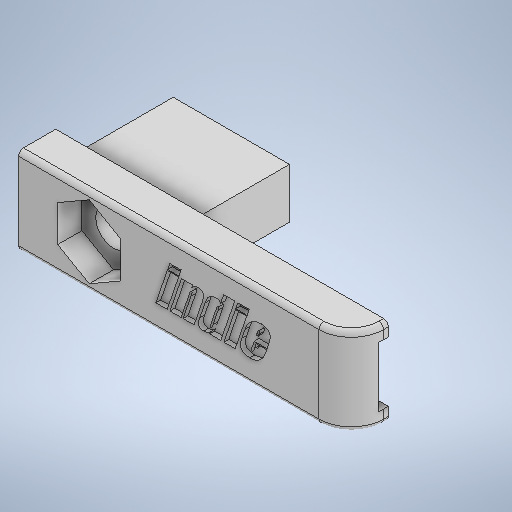
# Autodesk Inventor part: stereotax_holder_side
Saved by Autodesk Inventor 2025 (Build 290162000, 162)
## iProperties
Created: 2023-10-03
Part Number: stereotax_holder_side
Material: Generic
Document SubType Name: Modeling
Designer: mmelin
Density: 1 g/cm^3
Appearance: Default
Author: mmelin
Autodesk Inventor part; units mm, degrees
ref_plane "YZ Plane" through (0, 0, 0) normal (1, 0, 0) x (0, 1, 0)
ref_plane "XZ Plane" through (0, 0, 0) normal (0, 1, 0) x (-1, 0, 0)
ref_plane "XY Plane" through (0, 0, 0) normal (0, 0, 1) x (1, 0, 0)
sketch "Sketch1" plane through (0, 0, 0) normal (0, 0, 1) x (1, 0, 0)
  line L0 (-6.6, -4.4) -> (-23.2373, -4.4) projected
  line L1 (-23.2373, 1) -> (-6.6, 1) projected
  line L2 (-4.6226, -4.4) -> (-25.2226, -4.4)
  line L3 (-25.2226, -4.4) -> (-25.2226, 1)
  line L4 (-25.2226, 1) -> (-4.6226, 1)
  line L5 (-4.6226, 1) -> (-4.6226, -4.4)
  line L6 (-11.6, -0.9) -> (-11.6, -3.4) projected
  line L7 (-4.6226, 0.16) -> (-4.6226, -3.56) projected
  line L8 (-4.6226, 0.16) -> (-15, 0.16) projected
  line L9 (-15, 0.16) -> (-15, -3.56) projected
  line L10 (-15, -3.56) -> (-4.6226, -3.56) projected
  point P0 (0, 0)
  dimension "d1" = 20.6
  dimension "d36" = 0
  constraints: 8 end point, 2 collinear, 2 parallel, 1 horizontal, 1 perpendicular
  measures "d1" distance between parallel lines of L3 L5
  measures "d36" distance between parallel lines of L7 L5
extrude "Extrusion1" add sketch "Sketch1" along normal blind 1.7
sketch "Sketch2" plane through (0, 0, 0) normal (0, 0, -1) x (-1, 0, 0)
  line L0 (4.6226, 0.16) -> (4.6226, -3.56) projected
  line L1 (4.6226, 0.16) -> (15, 0.16) projected
  line L2 (15, 0.16) -> (15, -3.56) projected
  line L3 (15, -3.56) -> (4.6226, -3.56) projected
  line L4 (25.2226, -4.4) -> (4.6226, -4.4) projected
  line L5 (25.2226, 1) -> (25.2226, -4.4) projected
  line L6 (8.5501, -0.0891) -> (8.5501, -3.1391) projected
  line L7 (25.2226, -4.4) -> (4.6226, -4.4) projected
  line L8 (4.6226, -4.4) -> (4.6226, 1) projected
  line L9 (4.6226, 1) -> (25.2226, 1) projected
  line L10 (25.2226, 1) -> (25.2226, -4.4) projected
  line L11 (11.8, -2.35) -> (15, -2.35) projected
  line L12 (11.8, -1.05) -> (11.8, -2.35) projected
  line L13 (15, -1.05) -> (11.8, -1.05) projected
  point P0 (0, 0)
extrude "Extrusion2" add sketch "Sketch2" along normal blind 0.6 contours L8 L9 L5 L4 L3 L2 L1 | L2 L11 L12 L13
fillet "Fillet1" radius 2 1 edges at (-4.6226, -1.7, 1.7)
sketch "Sketch4" plane through (0, 0, -0.6) normal (0, 0, -1) x (-1, 0, 0)
  line L0 (24.45, -3.25) -> (17.25, -3.25)
  line L1 (17.25, -3.25) -> (17.25, -0.15)
  line L2 (17.25, -0.15) -> (24.45, -0.15)
  line L3 (24.45, -0.15) -> (24.45, -3.25)
  line L4 (24.6, -3.4) -> (24.6, 0) projected
  line L5 (17.1, -3.4) -> (24.6, -3.4) projected
  line L6 (17.1, 0) -> (17.1, -3.4) projected
  line L7 (24.6, 0) -> (17.1, 0) projected
  circle A0 centre (20.85, -1.7) radius 1.1 projected
  circle A1 centre (20.85, -1.7) radius 1.1
  point P0 (0, 0)
  dimension "d14" = 0.15
  dimension "d15" = 0.15
  dimension "d16" = 0.15
  dimension "d17" = 0.15
  constraints: 8 end point, 2 parallel, 1 centre point, 1 coincident, 1 concentric, 1 horizontal, 1 perpendicular
  measures "d14" distance between parallel lines of L7 L2
  measures "d15" distance between parallel lines of L6 L1
  measures "d16" distance between parallel lines of L4 L3
  measures "d17" distance between parallel lines of L5 L0
extrude "Extrusion5" add sketch "Sketch4" along normal blind 6.5 contours L0 L1 L2 L3
sketch "Sketch6" plane through (0, 0, 1.7) normal (0, 0, 1) x (1, 0, 0)
  circle A0 centre (-20.85, -1.7) radius 1.1 projected
  circle A1 centre (-20.85, -1.7) radius 1.1
  point P0 (0, 0)
  constraints: 1 centre point, 1 coincident
extrude "Extrusion7" cut sketch "Sketch6" against normal up to surface (8.8 mm away)
sketch "Sketch7" plane through (0, 0, 1.7) normal (0, 0, 1) x (1, 0, 0)
  circle A0 centre (-20.85, -1.7) radius 1.1 projected
  line L0 (-18.9, -2.8258) -> (-20.85, -3.9517)
  line L1 (-20.85, -3.9517) -> (-22.8, -2.8258)
  line L2 (-22.8, -2.8258) -> (-22.8, -0.5742)
  line L3 (-22.8, -0.5742) -> (-20.85, 0.5517)
  line L4 (-20.85, 0.5517) -> (-18.9, -0.5742)
  line L5 (-18.9, -0.5742) -> (-18.9, -2.8258)
  point P0 (0, 0)
  dimension "d27" = 3.9
  constraints: 12 end point, 1 coincident, 1 vertical, 13 other
  measures "d27" distance between parallel lines of L5 L2
extrude "Extrusion8" cut sketch "Sketch7" against normal blind 1.5
fillet "Fillet2" radius 0.3 6 edges at (-15.9226, 1, 1.7) (-5.2084, 1, 1.1142) (-4.6226, 1, -0.45) (-15.9226, -4.4, 1.7) (-5.2084, -4.4, 1.1142) (-4.6226, -4.4, -0.45)
sketch "Sketch9" plane through (0, 0, 1.7) normal (0, 0, 1) x (1, 0, 0)
  line L0 (-16.8365, -0.3734) -> (-8.2904, -0.3734) construction
  line L1 (-8.2904, -0.3734) -> (-8.2904, -3.0273) construction
  line L2 (-8.2904, -3.0273) -> (-16.8365, -3.0273) construction
  line L3 (-16.8365, -3.0273) -> (-16.8365, -0.3734) construction
  line L4 (-15.3132, -0.819) -> (-16.0253, -2.9134)
  line L5 (-16.0253, -2.9134) -> (-16.726, -2.9134)
  line L6 (-16.726, -2.9134) -> (-16.0139, -0.819)
  line L7 (-16.0139, -0.819) -> (-15.3132, -0.819)
  line L8 (-15.1609, -0.3734) -> (-15.2923, -0.76)
  line L9 (-15.2923, -0.76) -> (-15.993, -0.76)
  line L10 (-15.993, -0.76) -> (-15.8616, -0.3734)
  line L11 (-15.8616, -0.3734) -> (-15.1609, -0.3734)
  line L12 (-14.4412, -0.819) -> (-14.5154, -1.0037)
  spline S0 degree 2 poles (-14.5154, -1.0037) (-14.4716, -0.9028) (-14.2203, -0.7828) (-14.0851, -0.7828) knots 0 0 0 1 2 2 2
  spline S1 degree 2 poles (-14.0851, -0.7828) (-13.9137, -0.7828) (-13.75, -0.9465) (-13.7709, -1.1884) (-13.8623, -1.4568) knots 0 0 0 1 2 3 3 3
  line L13 (-13.8623, -1.4568) -> (-14.3574, -2.9134)
  line L14 (-14.3574, -2.9134) -> (-15.0409, -2.9134)
  line L15 (-15.0409, -2.9134) -> (-14.5516, -1.474)
  spline S2 degree 2 poles (-14.5516, -1.474) (-14.4831, -1.2702) (-14.4792, -1.2055) (-14.5173, -1.2055) knots 0 0 0 1 2 2 2
  spline S3 degree 2 poles (-14.5173, -1.2055) (-14.5592, -1.2055) (-14.6106, -1.2836) (-14.6868, -1.5082) knots 0 0 0 1 2 2 2
  line L16 (-14.6868, -1.5082) -> (-15.1647, -2.9134)
  line L17 (-15.1647, -2.9134) -> (-15.8483, -2.9134)
  line L18 (-15.8483, -2.9134) -> (-15.1361, -0.819)
  line L19 (-15.1361, -0.819) -> (-14.4412, -0.819)
  line L20 (-11.8402, -0.3734) -> (-12.7047, -2.9134)
  line L21 (-12.7047, -2.9134) -> (-13.3882, -2.9134)
  line L22 (-13.3882, -2.9134) -> (-13.3387, -2.7649)
  spline S4 degree 2 poles (-13.3387, -2.7649) (-13.4035, -2.8525) (-13.6453, -2.9496) (-13.7595, -2.9496) knots 0 0 0 1 2 2 2
  spline S5 degree 2 poles (-13.7595, -2.9496) (-13.9137, -2.9496) (-14.087, -2.7859) (-14.0775, -2.5726) (-13.9994, -2.3422) knots 0 0 0 1 2 3 3 3
  line L23 (-13.9994, -2.3422) -> (-13.6757, -1.3921)
  spline S6 degree 2 poles (-13.6757, -1.3921) (-13.5958, -1.1522) (-13.4606, -0.9446) (-13.1731, -0.7828) (-13.015, -0.7828) knots 0 0 0 1 2 3 3 3
  spline S7 degree 2 poles (-13.015, -0.7828) (-12.8951, -0.7828) (-12.7199, -0.8723) (-12.7199, -0.9465) knots 0 0 0 1 2 2 2
  line L24 (-12.7199, -0.9465) -> (-12.5238, -0.3734)
  line L25 (-12.5238, -0.3734) -> (-11.8402, -0.3734)
  spline S8 degree 2 poles (-12.8608, -1.3616) (-12.8246, -1.2588) (-12.8341, -1.2055) (-12.8684, -1.2055) knots 0 0 0 1 2 2 2
  spline S9 degree 2 poles (-12.8684, -1.2055) (-12.9046, -1.2055) (-12.9446, -1.2512) (-12.9827, -1.3616) knots 0 0 0 1 2 2 2
  line L26 (-12.9827, -1.3616) -> (-13.3197, -2.3555)
  spline S10 degree 2 poles (-13.3197, -2.3555) (-13.3616, -2.4736) (-13.354, -2.5269) (-13.3235, -2.5269) knots 0 0 0 1 2 2 2
  spline S11 degree 2 poles (-13.3235, -2.5269) (-13.2854, -2.5269) (-13.2359, -2.4641) (-13.1807, -2.3003) knots 0 0 0 1 2 2 2
  line L27 (-13.1807, -2.3003) -> (-12.8608, -1.3616)
  line L28 (-11.0996, -0.819) -> (-11.8117, -2.9134)
  line L29 (-11.8117, -2.9134) -> (-12.5124, -2.9134)
  line L30 (-12.5124, -2.9134) -> (-11.8002, -0.819)
  line L31 (-11.8002, -0.819) -> (-11.0996, -0.819)
  line L32 (-10.9472, -0.3734) -> (-11.0786, -0.76)
  line L33 (-11.0786, -0.76) -> (-11.7793, -0.76)
  line L34 (-11.7793, -0.76) -> (-11.6479, -0.3734)
  line L35 (-11.6479, -0.3734) -> (-10.9472, -0.3734)
  line L36 (-9.8372, -1.9328) -> (-10.6369, -1.9328)
  line L37 (-10.6369, -1.9328) -> (-10.7759, -2.3403)
  spline S12 degree 2 poles (-10.7759, -2.3403) (-10.8197, -2.4717) (-10.812, -2.5269) (-10.7759, -2.5269) knots 0 0 0 1 2 2 2
  spline S13 degree 2 poles (-10.7759, -2.5269) (-10.7264, -2.5269) (-10.6616, -2.445) (-10.6121, -2.3003) knots 0 0 0 1 2 2 2
  line L38 (-10.6121, -2.3003) -> (-10.5112, -2.0014)
  line L39 (-10.5112, -2.0014) -> (-9.86, -2.0014)
  line L40 (-9.86, -2.0014) -> (-9.921, -2.1823)
  spline S14 degree 2 poles (-9.921, -2.1823) (-9.9876, -2.3746) (-10.1095, -2.5859) (-10.376, -2.8297) (-10.6978, -2.9496) (-10.9073, -2.9496) knots 0 0 0 1 2 3 4 4 4
  spline S15 degree 2 poles (-10.9073, -2.9496) (-11.1091, -2.9496) (-11.3814, -2.8316) (-11.488, -2.6221) (-11.4708, -2.3746) (-11.3909, -2.1423) knots 0 0 0 1 2 3 4 4 4
  line L41 (-11.3909, -2.1423) -> (-11.191, -1.5501)
  spline S16 degree 2 poles (-11.191, -1.5501) (-11.0977, -1.2779) (-10.8368, -0.9542) (-10.4331, -0.7828) (-10.2123, -0.7828) knots 0 0 0 1 2 3 3 3
  spline S17 degree 2 poles (-10.2123, -0.7828) (-9.9438, -0.7828) (-9.6582, -0.9903) (-9.6315, -1.3312) (-9.7344, -1.632) knots 0 0 0 1 2 3 3 3
  line L42 (-9.7344, -1.632) -> (-9.8372, -1.9328)
  line L43 (-10.3893, -1.5387) -> (-10.3494, -1.4207)
  spline S18 degree 2 poles (-10.3494, -1.4207) (-10.298, -1.2721) (-10.2999, -1.2055) (-10.3284, -1.2055) knots 0 0 0 1 2 2 2
  spline S19 degree 2 poles (-10.3284, -1.2055) (-10.3703, -1.2055) (-10.4065, -1.2569) (-10.4636, -1.4207) knots 0 0 0 1 2 2 2
  line L44 (-10.4636, -1.4207) -> (-10.5036, -1.5387)
  line L45 (-10.5036, -1.5387) -> (-10.3893, -1.5387)
  point P0 (0, 0)
  constraints: 2 other
emboss "Emboss1" sketch "Sketch9" operation cut depth 0.3 direction (0, 0, -1)
equation "\"d15\" = d14"
equation "\"d16\" = d14"
equation "\"d17\" = d14"
body "Solid1"
